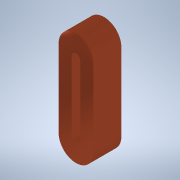
# Autodesk Inventor part: COILS
Saved by Autodesk Inventor 2022 (Build 260153000, 153)
## iProperties
Created: 2022-07-26
Part Number: COILS
Material: Copper
Document SubType Name: Modeling
Designer: Nathan Cai
Density: 8.94 g/cm^3
Appearance: Copper - Satin
Author: Nathan Cai
Autodesk Inventor part; units mm, degrees
ref_plane "YZ Plane" through (0, 0, 0) normal (1, 0, 0) x (0, 1, 0)
ref_plane "XZ Plane" through (0, 0, 0) normal (0, 1, 0) x (-1, 0, 0)
ref_plane "XY Plane" through (0, 0, 0) normal (0, 0, 1) x (1, 0, 0)
sketch "Sketch1" plane through (0, 0, 0) normal (0, 0, 1) x (1, 0, 0)
  line L0 (0, -5) -> (0, 5) construction
  line L1 (1, -5) -> (1, 5)
  line L2 (-1, 5) -> (-1, -5)
  arc A0 (-1, -5) -> (1, -5) centre (0, -5) ccw
  arc A1 (1, 5) -> (-1, 5) centre (0, 5) ccw
  line L3 (0, -6) -> (0, 6) construction
  line L4 (-4, -6) -> (-4, 6)
  line L5 (4, 6) -> (4, -6)
  arc A2 (-4, -6) -> (4, -6) centre (0, -6) ccw
  arc A3 (4, 6) -> (-4, 6) centre (0, 6) ccw
  point P0 (0, 0)
  dimension "d0" = 5
  dimension "d1" = 2
  dimension "d2" = 1
  dimension "d3" = 3
  constraints: 16 end point, 8 point on circle, 8 tangent, 4 centre point, 2 midpoint, 2 parallel, 1 point on line, 1 vertical
  measures "d0" distance of point (0, 0) L0.end
  measures "d1" diameter of A1
  measures "d2" distance of L0.end L3.end
  measures "d3" distance between parallel lines of L5 L1
extrude "Extrusion1" add sketch "Sketch1" along normal blind 6.5
body "Solid1"
